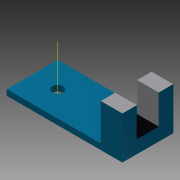
# Autodesk Inventor part: optical sensor pcb
Saved by Autodesk Inventor 2013 (Build 170138000, 138)
## iProperties
Created: 2012-12-12
Part Number: optical sensor pcb
Material: Generic
Document SubType Name: Modeling
Designer: Nico
Density: 1 g/cm^3
Author: Nico
Autodesk Inventor part; units mm, degrees
ref_plane "YZ Plane" through (0, 0, 0) normal (1, 0, 0) x (0, 1, 0)
ref_plane "XZ Plane" through (0, 0, 0) normal (0, 1, 0) x (-1, 0, 0)
ref_plane "XY Plane" through (0, 0, 0) normal (0, 0, 1) x (1, 0, 0)
sketch "Sketch1" plane through (0, 0, 0) normal (0, 0, 1) x (1, 0, 0)
  line L0 (0.4379, 0) -> (32.5379, 0)
  line L1 (32.5379, 0) -> (32.5379, 14.1)
  line L2 (32.5379, 14.1) -> (0.4379, 14.1)
  line L3 (0.4379, 14.1) -> (0.4379, 0)
  circle A0 centre (7.5379, 7.05) radius 1.5
  point P0 (0, 0)
  dimension "d0" = 14.1
  dimension "d2" = 32.1
  dimension "d3" = 3
  dimension "d4" = 7.1
  dimension "d5" = 7.05
  constraints: 8 end point, 2 parallel, 1 centre point, 1 horizontal, 1 perpendicular
  measures "d0" distance of L2.end L0.start
  measures "d2" distance of L0.start L0.end
  measures "d3" diameter of A0
  measures "d4" distance from line of L3 A0.centre
  measures "d5" distance from line of A0.centre L2
extrude "Extrusion1" add sketch "Sketch1" along normal blind 1.6
sketch "Sketch2" plane through (0, 0, 1.6) normal (0, 0, 1) x (1, 0, 0)
  line L0 (0.4379, 0) -> (32.5379, 0) projected
  line L1 (26.5379, 0) -> (32.5379, 0)
  line L2 (32.5379, 0) -> (32.5379, 14.1)
  line L3 (32.5379, 14.1) -> (26.5379, 14.1)
  line L4 (26.5379, 14.1) -> (26.5379, 0)
  point P0 (0, 0)
  dimension "d8" = 6
  constraints: 8 end point, 2 parallel, 1 horizontal, 1 perpendicular, 1 point on line
  measures "d8" distance between parallel lines of L2 L4
extrude "Extrusion2" add sketch "Sketch2" along normal blind 2
sketch "Sketch3" plane through (0, 0, 3.6) normal (0, 0, 1) x (1, 0, 0)
  line L0 (26.5379, 0) -> (32.5379, 0) projected
  line L1 (32.5379, 0) -> (32.5379, 14.1) projected
  line L2 (26.5379, 14.1) -> (32.5379, 14.1)
  line L3 (32.5379, 14.1) -> (32.5379, 10.1)
  line L4 (32.5379, 10.1) -> (26.5379, 10.1)
  line L5 (26.5379, 10.1) -> (26.5379, 14.1)
  line L6 (26.5379, 0) -> (32.5379, 0)
  line L7 (32.5379, 0) -> (32.5379, 4)
  line L8 (32.5379, 4) -> (26.5379, 4)
  line L9 (26.5379, 4) -> (26.5379, 0)
  point P0 (0, 0)
  dimension "d12" = 4
  dimension "d14" = 4
  constraints: 16 end point, 4 parallel, 2 horizontal, 2 perpendicular, 2 point on line
  measures "d12" distance between parallel lines of L4 L2
  measures "d14" distance between parallel lines of L8 L0
extrude "Extrusion3" add sketch "Sketch3" along normal blind 8.2
body "Solid1"
